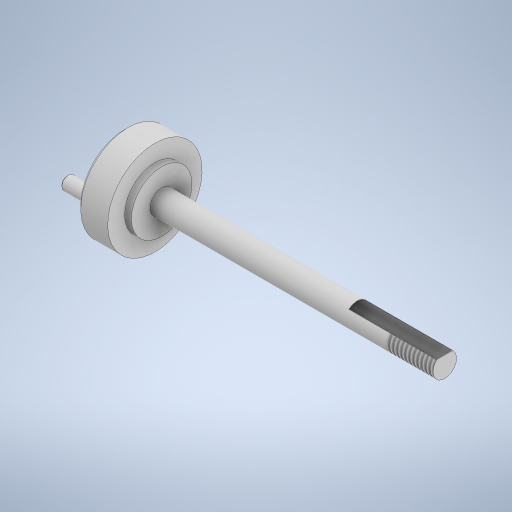
# Autodesk Inventor part: Hudson 1-62A
Saved by Autodesk Inventor 2024.2 (Build 282272000, 272)
## iProperties
Created: 2024-10-07
Part Number: Hudson 1-62A
Material: Genérico
Document SubType Name: Modeling
Designer: Monica Mora
Density: 1 g/cm^3
Appearance: Valor por defecto
Author: Monica Mora
Autodesk Inventor part; units mm, degrees
ref_plane "YZ Plane" through (0, 0, 0) normal (1, 0, 0) x (0, 1, 0)
ref_plane "XZ Plane" through (0, 0, 0) normal (0, 1, 0) x (-1, 0, 0)
ref_plane "XY Plane" through (0, 0, 0) normal (0, 0, 1) x (1, 0, 0)
sketch "Boceto1" plane through (0, 0, 0) normal (0, 0, 1) x (1, 0, 0)
  line L0 (0, 0) -> (47.5, 0)
  line L1 (0, 0) -> (0, 7)
  line L2 (0, 7) -> (4.5, 7)
  line L3 (4.5, 7) -> (4.5, 0)
  line L4 (4.5, 4.5) -> (5.5, 4.5)
  line L5 (5.5, 4.5) -> (5.5, 0)
  line L6 (0, 1.75) -> (47.5, 1.75)
  line L7 (47.5, 1.75) -> (47.5, 0)
  line L8 (4.4935, -4.5) -> (-8.5065, -4.5)
  line L9 (4.4935, -3.5) -> (-8.5065, -3.5)
  line L10 (-8.5065, -3.5) -> (-8.5065, -4.5)
  line L11 (4.4935, -3.5) -> (4.4935, -4.5)
  line L12 (40.5, 1.75) -> (40.5, 0)
  point P0 (5.5, 1.75)
  dimension "d0" = 14
  dimension "d1" = 3.5
  dimension "d2" = 4.5
  dimension "d3" = 1
  dimension "d4" = 9
  dimension "d5" = 43
  dimension "d6" = 4.5
  dimension "d7" = 2
  dimension "d8" = 13
  dimension "d33" = 7
  constraints: 26 end point, 7 perpendicular, 6 point on line, 4 horizontal, 1 parallel, 1 vertical
  measures "d0" diameter of L2 L0
  measures "d1" diameter of L6 L0
  measures "d2" distance of L1.end L2.end
  measures "d3" distance of L4.start L4.end
  measures "d4" diameter of L4 L0
  measures "d5" distance between parallel lines of L3 L7
  measures "d6" distance between parallel lines of L8 L0
  measures "d7" diameter of L9 L8
  measures "d8" distance of L8.start L8.end
  measures "d33" distance between parallel lines of L7 L12
revolve "Revolución1" add sketch "Boceto1" angle 360 about axis through (0, 0, 0) along (1, 0, 0) contours L1 L6 L3 L0 | L3 L6 L5 L0 | L1 L2 L3 L6 | L5 L6 L12 L0 | L3 L4 L5 L6 | L12 L6 L7 L0
revolve "Revolución2" add sketch "Boceto1" angle 360 about axis through (4.4935, -4.5, 0) along (-1, 0, 0) contours L8 L10 L9 L11
shell "Vaciado1" thickness 1 removed faces 0
sketch "Boceto2" plane through (0, 0, 0) normal (-1, 0, 0) x (0, 0, 1)
  circle A0 centre (0, 0) radius 1.75 projected
  constraints: 1 coincident
hole "Agujero1" at (0, 0, 0) direction (1, 0, 0) diameter 3.4 depth 47.4
thread "Rosca1" size "M3.5x0.6" class "6g" standard "ANSI Metric M Profile" length 7
sketch "Boceto3" plane through (0, 0, 0) normal (0, 0, 1) x (1, 0, 0)
  line L0 (4.5, -7) -> (0, -7) projected
  line L1 (0, -7) -> (0, -5.5) projected
  line L2 (0, -5.5) -> (-8.5065, -5.5) projected
  line L3 (-8.5065, -5.5) -> (-8.5065, -3.5) projected
  line L4 (-8.5065, -3.5) -> (0, -3.5) projected
  line L5 (0, -3.5) -> (0, -1.7) projected
  line L6 (0, -1.7) -> (1, -1.7) projected
  line L7 (1, -1.7) -> (1, -6) projected
  line L8 (1, -6) -> (3.5, -6) projected
  line L9 (3.5, -6) -> (3.5, -3.5) projected
  line L10 (3.5, -3.5) -> (4.5, -3.5) projected
  line L11 (4.5, -3.5) -> (4.5, -1.7) projected
  line L12 (4.5, -1.7) -> (47.4, -1.7) projected
  line L13 (47.4, -1.7) -> (47.4, 1.7) projected
  line L14 (47.4, 1.7) -> (4.5, 1.7) projected
  line L15 (4.5, 1.7) -> (4.5, 3.5) projected
  line L16 (4.5, 3.5) -> (3.5, 3.5) projected
  line L17 (3.5, 3.5) -> (3.5, 6) projected
  line L18 (3.5, 6) -> (1, 6) projected
  line L19 (1, 6) -> (1, 1.7) projected
  line L20 (1, 1.7) -> (0, 1.7) projected
  line L21 (0, 1.7) -> (0, 7) projected
  line L22 (0, 7) -> (4.5, 7) projected
  line L23 (4.5, 7) -> (4.5, 4.5) projected
  line L24 (4.5, 4.5) -> (5.5, 4.5) projected
  line L25 (5.5, 4.5) -> (5.5, 1.75) projected
  line L26 (5.5, 1.75) -> (47.5, 1.75) projected
  line L27 (47.5, 1.75) -> (47.5, -1.75) projected
  line L28 (47.5, -1.75) -> (5.5, -1.75) projected
  line L29 (5.5, -1.75) -> (5.5, -4.5) projected
  line L30 (5.5, -4.5) -> (4.5, -4.5) projected
  line L31 (4.5, -4.5) -> (4.5, -7) projected
  line L32 (47.5, 1.25) -> (34.5, 1.25)
  line L33 (34.5, 1.25) -> (34.5, 3.25)
  line L34 (34.5, 3.25) -> (47.5, 3.25)
  line L35 (47.5, 3.25) -> (47.5, 1.25)
  point P0 (0, 0)
  dimension "d22" = 0.5
  dimension "d23" = 13
  dimension "d24" = 2
  constraints: 8 end point, 2 parallel, 1 horizontal, 1 perpendicular, 1 point on line
  measures "d22" distance between parallel lines of L26 L32
  measures "d23" distance of L33.end L34.end
  measures "d24" distance of L32.end L33.end
extrude "Extrusión1" cut sketch "Boceto3" along normal through all both and the other way through all contours L32 L13 L14 L33 L26 L27 | L26 L33 L34 L35 | L32 L33 L14 L13
chamfer "Chaflán1" distance 0.5 angle 45 1 edges at (0, -7, 0)
chamfer "Chaflán2" distance 0.2 angle 45 1 edges at (-8.5065, -5.5, 0)
